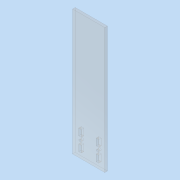
# Autodesk Inventor part: bed
Saved by Autodesk Inventor 2016 SP1 (Build 200210100, 210)
## iProperties
Created: 2016-03-25
Part Number: bed
Material: Acrylic, Clear
Document SubType Name: Modeling
Designer: Mohamed A.
Density: 1.19 g/cm^3
Appearance: Transparent - Clear
Mass: 19.021 g
Surface Area: 117.42 cm^2
Volume: 15.984 cm^3
Author: Mohamed A.
Autodesk Inventor part; units mm, degrees
ref_plane "YZ Plane" through (0, 0, 0) normal (1, 0, 0) x (0, 1, 0)
ref_plane "XZ Plane" through (0, 0, 0) normal (0, 1, 0) x (-1, 0, 0)
ref_plane "XY Plane" through (0, 0, 0) normal (0, 0, 1) x (1, 0, 0)
sketch "Sketch2" plane through (0, 0, 0) normal (0, 1, 0) x (-1, 0, 0)
  line L0 (8.5, 37) -> (-8.5, 37)
  line L1 (-8.5, 37) -> (-8.5, -37)
  line L2 (-8.5, -37) -> (8.5, -37)
  line L3 (8.5, -37) -> (8.5, 37)
  line L4 (8.5, 37) -> (-8.5, -37) construction
  line L5 (-8.5, 37) -> (8.5, -37) construction
  line L6 (18.5, 47) -> (-18.5, 47)
  line L7 (-18.5, 47) -> (-18.5, -47)
  line L8 (-18.5, -47) -> (18.5, -47)
  line L9 (18.5, -47) -> (18.5, 47)
  line L10 (18.5, -47) -> (-18.5, -47)
  line L11 (-18.5, -47) -> (-18.5, -97)
  line L12 (-18.5, -97) -> (18.5, -97)
  line L13 (18.5, -97) -> (18.5, -47)
  point P0 (0, 0)
  dimension "d0" = 17
  dimension "d1" = 74
  dimension "d2" = 10
  dimension "d5" = 50
  constraints: 28 end point, 6 parallel, 3 perpendicular, 2 horizontal, 2 midpoint, 1 collinear, 3 other
  measures "d0" distance of L2.end L1.end
  measures "d1" distance of L1.end L0.end
  measures "d2" distance between parallel lines of L3 L9
  measures "d5" distance of L11.end L10.end
extrude "Extrusion1" add sketch "Sketch2" along normal blind 3 contours L3 L2 L1 L0 | L9 L8 L7 L6 | L13 L12 L11 L8
sketch "Sketch3" plane through (0, 3, 0) normal (0, 1, 0) x (1, 0, 0)
  line L0 (8.5, 67.8333) -> (8.5, 75.5) projected
  line L1 (8.5, 67.8333) -> (11.5, 67.8333) projected
  line L2 (11.5, 75.5) -> (11.5, 67.8333) projected
  line L3 (8.5, 75.5) -> (11.5, 75.5) projected
  line L4 (8.5, 83.5) -> (8.5, 91.1667) projected
  line L5 (8.5, 83.5) -> (11.5, 83.5) projected
  line L6 (11.5, 91.1667) -> (11.5, 83.5) projected
  line L7 (8.5, 91.1667) -> (11.5, 91.1667) projected
  line L8 (-11.5, 83.5) -> (-11.5, 91.1667) projected
  line L9 (-11.5, 83.5) -> (-8.5, 83.5) projected
  line L10 (-8.5, 91.1667) -> (-8.5, 83.5) projected
  line L11 (-11.5, 91.1667) -> (-8.5, 91.1667) projected
  line L12 (-11.5, 67.8333) -> (-11.5, 75.5) projected
  line L13 (-11.5, 67.8333) -> (-8.5, 67.8333) projected
  line L14 (-8.5, 75.5) -> (-8.5, 67.8333) projected
  line L15 (-11.5, 75.5) -> (-8.5, 75.5) projected
  line L16 (8.5, 75.5) -> (11.5, 83.5) construction
  line L17 (11.5, 75.5) -> (8.5, 83.5) construction
  line L18 (-8.5, 75.5) -> (-11.5, 83.5) construction
  line L19 (-11.5, 75.5) -> (-8.5, 83.5) construction
  circle A0 centre (-10, 79.5) radius 1.35
  circle A1 centre (10, 79.5) radius 1.35
  point P0 (0, 0)
  dimension "d6" = 2.7
  dimension "d7" = 2.7
  constraints: 8 end point, 2 centre point, 2 midpoint, 2 parallel
  measures "d6" diameter of A0
  measures "d7" diameter of A1
extrude "Extrusion2" cut sketch "Sketch3" against normal blind 3
body "Solid1"
